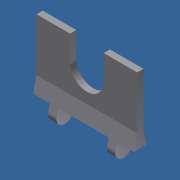
# Autodesk Inventor part: kinect bracket
Saved by Autodesk Inventor 2012 (Build 160160000, 160)
## iProperties
Created: 2012-10-30
Part Number: kinect bracket
Material: Default
Document SubType Name: Modeling
Designer: Ed
Density: 1 g/cm^3
Author: Ed
Autodesk Inventor part; units mm, degrees
ref_plane "YZ Plane" through (0, 0, 0) normal (1, 0, 0) x (0, 1, 0)
ref_plane "XZ Plane" through (0, 0, 0) normal (0, 1, 0) x (-1, 0, 0)
ref_plane "XY Plane" through (0, 0, 0) normal (0, 0, 1) x (1, 0, 0)
sketch "Sketch1" plane through (0, 0, 0) normal (0, 0, 1) x (1, 0, 0)
  line L0 (-6.8944, -9.4305) -> (69.3056, -9.4305)
  line L1 (69.3056, -9.4305) -> (69.3056, 41.3695)
  line L2 (69.3056, 41.3695) -> (-6.8944, 41.3695)
  line L3 (-6.8944, 41.3695) -> (-6.8944, -9.4305)
  line L4 (18.5056, 41.3695) -> (43.9056, 41.3695)
  line L5 (43.9056, 41.3695) -> (43.9056, 22.3195)
  line L6 (43.9056, 22.3195) -> (18.5056, 22.3195)
  line L7 (18.5056, 22.3195) -> (18.5056, 41.3695)
  arc A0 (18.5056, 22.3195) -> (43.9056, 22.3195) centre (31.2056, 22.3195) ccw
  point P0 (0, 0)
  point P1 (14.7078, 41.3695)
  point P2 (47.7034, 41.3695)
  point P3 (31.2056, 41.3695)
  dimension "d0" = 76.2
  dimension "d1" = 50.8
  dimension "d6" = 25.4
  dimension "d7" = 19.05
  constraints: 16 end point, 4 parallel, 3 point on line, 2 horizontal, 2 midpoint, 2 perpendicular, 2 point on circle, 2 tangent, 1 centre point
  measures "d0" distance of L0.start L0.end
  measures "d1" distance of L2.end L0.start
  measures "d6" distance of L5.end L6.end
  measures "d7" distance of L4.end L5.end
extrude "Extrusion2" add sketch "Sketch1" along normal blind 4.7625 contours L3 L2 L7 A0 L5 L1 L0
sketch "Sketch2" plane through (69.3056, -9.4305, 0) normal (1, 0, 0) x (0, 0, -1)
  line L0 (-4.7625, 50.8) -> (-4.7625, 0) projected
  line L1 (0, 0) -> (-4.7625, 0) projected
  line L2 (0, 0) -> (0, 50.8) projected
  line L3 (0, 50.8) -> (-4.7625, 50.8) projected
  circle A0 centre (-2.3813, -6.35) radius 6.35
  line L4 (3.7948, -4.8737) -> (0, 11.0013)
  line L5 (-8.5573, -4.8737) -> (-4.7625, 11.0013)
  point P0 (0, 9.4305)
  point P1 (-2.3813, 0)
  dimension "d10" = 12.7
  dimension "d11" = 15.875
  constraints: 4 end point, 3 tangent, 2 point on circle, 2 point on line, 1 centre point, 1 equal length, 1 midpoint, 1 vertical alignment
  measures "d10" diameter of A0
  measures "d11" vertical distance of L4.start L4.end
extrude "Extrusion3" add sketch "Sketch2" against normal up to surface (76.2 mm away) contours L0 L1 A0 L5 | A0 | L4 A0 L1 L2
sketch "Sketch3" plane through (0, 0, 4.7625) normal (0, 0, 1) x (1, 0, 0)
  arc A0 (18.5056, 22.3195) -> (43.9056, 22.3195) centre (31.2056, 22.3195) ccw projected
  line L0 (56.6056, -9.4305) -> (56.6056, -22.1305)
  line L1 (5.8056, -22.1305) -> (5.8056, -9.4305)
  line L2 (69.3056, -9.4305) -> (69.3056, -22.1305)
  line L3 (-6.8944, -22.1305) -> (-6.8944, -9.4305)
  line L4 (5.8056, -22.1305) -> (-6.8944, -22.1305)
  line L5 (-6.8944, -9.4305) -> (5.8056, -9.4305)
  line L6 (56.6056, -9.4305) -> (69.3056, -9.4305)
  line L7 (69.3056, -22.1305) -> (56.6056, -22.1305)
  line L8 (12.1556, -9.4305) -> (50.2556, -9.4305)
  line L9 (50.2556, -9.4305) -> (50.2556, -22.1305)
  line L10 (50.2556, -22.1305) -> (12.1556, -22.1305)
  line L11 (12.1556, -22.1305) -> (12.1556, -9.4305)
  point P0 (0, 0)
  point P1 (31.2056, 9.6195)
  point P2 (31.2056, -9.4305)
  dimension "d14" = 50.8
  dimension "d18" = 76.2
  dimension "d19" = 6.35
  dimension "d20" = 6.35
  dimension "d21" = 12.7
  dimension "d22" = 19.05
  constraints: 24 end point, 8 parallel, 5 collinear, 3 horizontal, 3 perpendicular, 1 midpoint, 1 point on circle, 1 vertical alignment
  measures "d14" distance between parallel lines of L0 L1
  measures "d18" distance between parallel lines of L2 L3
  measures "d19" distance between parallel lines of L11 L1
  measures "d20" distance between parallel lines of L0 L9
  measures "d21" distance of L2.start L2.end
  measures "d22" distance from line of point (31.206, 9.62) L8
extrude "Extrusion4" cut sketch "Sketch3" along normal through all both and the other way through all
body "Solid2"
